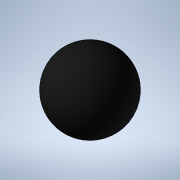
# Autodesk Inventor part: 2200 Ball
Saved by Autodesk Inventor 2021 (Build 250183000, 183)
## iProperties
Created: 2026-07-02
Part Number: 2200 Ball
Material: Generic
Catalog Web Link: www.3dfindit.com
Description: cylindrical_bore_B-
Vendor: NSK_RB
Document SubType Name: Modeling
Designer: psAdmin
Manufacturer: NSK_RB
Mass: 0.0535468 g
Surface Area: 0.687026 cm^2
Volume: 0.0535468 cm^3
Density: 1 g/cm^3
Appearance: PSOLRGB-128-128-128
Category: PARTsolutions
Company: NSK_RB
Title: 2200 Ball
Author: Cadenas PARTsolutions
PSOL_IDENT_0: {$CADENAS_DATA/23d-libs/nsk_rb/roller_bearings/self_aliging_bb/cylindrical_bore_b.prj},171 {VTYP=3D}
PSOL_IDENT_1: ,{NB=2200 Ball},{LINA=2200 Ball},{NN=cylindrical_bore_B},{DATE=06.08.2025 00:27:17},{GEOMDATE=14.01.
PSOL_IDENT_2: 2008 00:00:00},{VERSION=},{LINEID=120},{WBVAR=},{WBNUMERIC=}  {NB=2200 Ball},{LINA=2200 Ball},{KT=DU
PSOL_IDENT_3: MMY},{IDNR=},{STAN=},{ORDER=2200},{SD=10},{X=10},{D=30},{DD=30},{B=14},{R=0.6},{SDE1=22.420},{DI1=15
PSOL_IDENT_4: .20},{CR1=7450},{COR1=1590},{CR2=760},{COR2=162},{LG=24000},{LO=28000},{DA1=14.0},{DA2=26.0},{RA=0.6
PSOL_IDENT_5: },{E=0.64},{Y2=1.5},{Y3=0.98},{Y0=1.00},{MASS=0.042},{SC=1}
NB: 2200 Ball
NN: cylindrical_bore_B
NBSYN: $ORDER. Ball
LINA: 2200 Ball
CATALOG: NSK Rolling Bearing
ORDER: 2200
SD: 10
X: 10
D: 30
DD: 30
B: 14
R: 0.6
SDE1: 22.42
DI1: 15.2
CR1: 7450
COR1: 1590
CR2: 760
COR2: 162
LG: 24000
LO: 28000
DA1: 14
DA2: 26
RA: 0.6
E: 0.64
Y2: 1.5
Y3: 0.98
Y0: 1
MASS: 0.042
SC: 1
SUPPLIER: NSK_RB
ARTICLENO: 2200 Ball
BOMINFO: 2200 Ball
CREATOR: CADENAS GmbH
Autodesk Inventor part; units mm, degrees
sketch "Sketch_1" plane through (0, 0, 0) normal (0, 0, 1) x (1, 0, 0)
  line L0 (2.3382, 0) -> (-2.3382, 0)
  arc A0 (2.3382, 0) -> (-2.3382, 0) centre (0, 0) ccw
  line L1 (2.3382, 0) -> (-2.3382, 0)
  constraints: 4 end point, 2 point on circle, 1 centre point
revolve "Revolution1" add sketch "Sketch_1" angle 360 about axis through (2.3382, 0, 0) along (1, 0, 0)
ref_plane "ip_cb_1_XY" through (0, 0, 0) normal (-1, 0, 0) x (0, 0, -1)
ref_plane "ip_cb_1_YZ" through (0, 0, 0) normal (0, 0, -1) x (0, -1, 0)
ref_plane "ip_cb_1_ZX" through (0, 0, 0) normal (0, -1, 0) x (-1, 0, 0)
body "Solid1"
